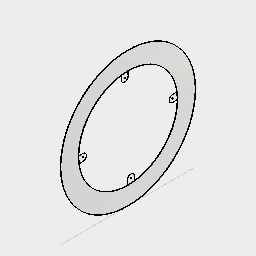
base (Autodesk Fusion 360 design; units mm, degrees)
Autodesk Fusion 360 part; units mm, degrees
note: some values were not read from the file. Set by a fixed rule: which sketch regions a step uses.
sketch "Sketch1" plane through (0, 0, 0) normal (1, 0, 0) x (0, 0, -1)
  circle A0 centre (0, 0) radius 381
  circle A1 centre (0, 0) radius 330.2
  dimension "d1" = 762
  dimension "d2" = 660.4
  measures "d1" diameter of A0
  measures "d2" diameter of A1
sketch "Sketch1 (2)" plane through (0, 0, 0) normal (1, 0, 0) x (0, 0, -1) in component "outer ring"
  circle A0 centre (0, 0) radius 381
  circle A1 centre (0, 0) radius 368.3
  dimension "d15" = 762
  dimension "d16" = 736.6
  measures "d15" diameter of A0
  measures "d16" diameter of A1
extrude "Extrude1" add sketch "Sketch1 (2)" along normal blind 6.35 makes body 1 in component "outer ring"
sketch "Sketch1 (3)" plane through (0, 0, 0) normal (1, 0, 0) x (0, 0, -1) in component "Top"
  circle A0 centre (0, 0) radius 381
  circle A1 centre (0, 0) radius 330.2
  dimension "d19" = 762
  dimension "d20" = 660.4
  measures "d19" diameter of A0
  measures "d20" diameter of A1
extrude "Extrude1'" add sketch "Sketch1 (3)" along normal blind 3.175 separate body makes body 2 in component "Top"
sketch "Sketch1 (4)" plane through (0, 0, 0) normal (1, 0, 0) x (0, 0, -1) in component "magnets"
  line L0 (-82.7081, 358.8931) -> (-70.2852, 361.5313)
  line L1 (-70.2852, 361.5313) -> (-67.647, 349.1083)
  line L2 (-67.647, 349.1083) -> (-80.0699, 346.4701)
  line L3 (-80.0699, 346.4701) -> (-82.7081, 358.8931)
  circle A0 centre (0, 0) radius 368.3
  line L4 (-82.7081, 358.8931) -> (-70.2852, 361.5313)
  dimension "d23" = 12.7
  dimension "d24" = 12.7
  measures "d23" distance of L0.start L0.end
  measures "d24" distance of L0.start L2.end
extrude "Extrude1''" add sketch "Sketch1 (4)" along normal blind 6.35 separate body contours L0 L1 L2 L3 L4 makes body 3 in component "magnets"
pattern_circular "C-Pattern1" count 176 over 360 about axis through (6.35, 0, 0) along (-1, 0, 0) of bodies 3 makes body 4 at (0, 358.1778, 64.9449) makes body 5 at (0, 356.6562, 47.3444) makes body 6 at (0, 358.1187, 34.5844) makes body 7 at (0, 363.0678, 26.2854) makes body 8 at (0, 363.7747, 13.3099) makes body 9 at (0, 364.0179, 0.3174) makes body 10 at (0, 363.7973, -12.6754) makes body 11 at (0, 363.1131, -25.6521) makes body 12 at (0, 357.286, -42.3296) makes body 13 at (0, 360.3579, -51.4909) makes body 14 at (0, 353.356, -67.7102) makes body 15 at (0, 350.7141, -80.2792) makes body 16 at (0, 347.6253, -92.7458) makes body 17 at (0, 344.0934, -105.0943) makes body 18 at (0, 340.1231, -117.3088) makes body 19 at (0, 341.1774, -126.9138) makes body 20 at (0, 336.4302, -139.0104) makes body 21 at (0, 325.6346, -152.9942) makes body 22 at (0, 319.9664, -164.5194) makes body 23 at (0, 319.643, -174.1766) makes body 24 at (0, 313.2226, -185.4744) makes body 25 at (0, 300.5468, -197.7796) makes body 26 at (0, 299.1929, -207.3469) makes body 27 at (0, 291.6016, -217.8937) makes body 28 at (0, 277.683, -228.7733) makes body 29 at (0, 269.3407, -238.5387) makes body 30 at (0, 260.655, -248.0001) makes body 31 at (0, 257.624, -257.1751) makes body 32 at (0, 242.2988, -265.9632) makes body 33 at (0, 238.621, -274.8985) makes body 34 at (0, 222.7078, -282.5709) makes body 35 at (0, 218.4019, -291.2211) makes body 36 at (0, 207.8684, -298.8309) makes body 37 at (0, 191.2263, -304.7583) makes body 38 at (0, 186.0204, -312.8986) makes body 39 at (0, 174.7338, -319.3388) makes body 40 at (0, 157.5535, -323.4533) makes body 41 at (0, 145.9083, -328.8706) makes body 42 at (0, 134.0772, -333.8689) makes body 43 at (0, 127.5087, -340.9556) makes body 44 at (0, 115.2579, -345.2894) makes body 45 at (0, 97.62, -346.2881) makes body 46 at (0, 90.3316, -352.6321) makes body 47 at (0, 72.6674, -352.3699) makes body 48 at (0, 64.9449, -358.1778) makes body 49 at (0, 47.3444, -356.6562) makes body 50 at (0, 39.2274, -361.8983) makes body 51 at (0, 26.2854, -363.0678) makes body 52 at (0, 13.3099, -363.7747) makes body 53 at (0, -3.8949, -359.7637) makes body 54 at (0, -12.6754, -363.7973) makes body 55 at (0, -25.6521, -363.1131) makes body 56 at (0, -42.3296, -357.286) makes body 57 at (0, -51.4909, -360.3579) makes body 58 at (0, -64.3202, -358.2905) makes body 59 at (0, -77.0674, -355.7665) makes body 60 at (0, -92.7458, -347.6253) makes body 61 at (0, -102.2511, -349.3621) makes body 62 at (0, -117.3088, -340.1231) makes body 63 at (0, -129.3739, -335.7194) makes body 64 at (0, -141.2741, -330.8878) makes body 65 at (0, -152.9942, -325.6346) makes body 66 at (0, -162.6568, -325.6561) makes body 67 at (0, -175.8349, -313.8904) makes body 68 at (0, -185.4744, -313.2226) makes body 69 at (0, -197.7796, -300.5468) makes body 70 at (0, -208.3808, -293.296) makes body 71 at (0, -218.7164, -285.6716) makes body 72 at (0, -228.1628, -283.6387) makes body 73 at (0, -238.5387, -269.3407) makes body 74 at (0, -247.816, -266.639) makes body 75 at (0, -257.1751, -257.624) makes body 76 at (0, -266.2064, -248.2807) makes body 77 at (0, -274.4419, -232.6516) makes body 78 at (0, -282.5709, -222.7078) makes body 79 at (0, -290.3398, -212.4803) makes body 80 at (0, -298.8309, -207.8684) makes body 81 at (0, -304.7583, -191.2263) makes body 82 at (0, -311.3894, -180.227) makes body 83 at (0, -317.6237, -168.9979) makes body 84 at (0, -323.4533, -157.5535) makes body 85 at (0, -330.9905, -151.5073) makes body 86 at (0, -336.1872, -139.5969) makes body 87 at (0, -338.4417, -122.0752) makes body 88 at (0, -345.2894, -115.2579) makes body 89 at (0, -346.2881, -97.62) makes body 90 at (0, -352.6321, -90.3316) makes body 91 at (0, -352.3699, -72.6674) makes body 92 at (0, -358.1778, -64.9449) makes body 93 at (0, -356.6562, -47.3444) makes body 94 at (0, -361.8983, -39.2274) makes body 95 at (0, -363.0678, -26.2854) makes body 96 at (0, -363.7747, -13.3099) makes body 97 at (0, -364.0179, -0.3174) makes body 98 at (0, -363.7973, 12.6754) makes body 99 at (0, -363.1131, 25.6521) makes body 100 at (0, -361.9662, 38.5961) makes body 101 at (0, -360.3579, 51.4909) makes body 102 at (0, -358.2905, 64.3202) makes body 103 at (0, -350.7141, 80.2792) makes body 104 at (0, -347.6253, 92.7458) makes body 105 at (0, -349.3621, 102.2511) makes body 106 at (0, -345.4899, 114.6555) makes body 107 at (0, -341.1774, 126.9138) makes body 108 at (0, -330.8878, 141.2741) makes body 109 at (0, -325.6346, 152.9942) makes body 110 at (0, -325.6561, 162.6568) makes body 111 at (0, -319.643, 174.1766) makes body 112 at (0, -313.2226, 185.4744) makes body 113 at (0, -306.403, 196.5359) makes body 114 at (0, -299.1929, 207.3469) makes body 115 at (0, -285.6716, 218.7164) makes body 116 at (0, -283.6387, 228.1628) makes body 117 at (0, -275.3143, 238.1412) makes body 118 at (0, -260.655, 248.0001) makes body 119 at (0, -251.6372, 257.1455) makes body 120 at (0, -242.2988, 265.9632) makes body 121 at (0, -238.621, 274.8985) makes body 122 at (0, -228.6571, 283.2403) makes body 123 at (0, -218.4019, 291.2211) makes body 124 at (0, -207.8684, 298.8309) makes body 125 at (0, -191.2263, 304.7583) makes body 126 at (0, -186.0204, 312.8986) makes body 127 at (0, -174.7338, 319.3388) makes body 128 at (0, -157.5535, 323.4533) makes body 129 at (0, -151.5073, 330.9905) makes body 130 at (0, -134.0772, 333.8689) makes body 131 at (0, -127.5087, 340.9556) makes body 132 at (0, -115.2579, 345.2894) makes body 133 at (0, -97.62, 346.2881) makes body 134 at (0, -90.3316, 352.6321) makes body 135 at (0, -77.6878, 355.6315) makes body 136 at (0, -64.9449, 358.1778) makes body 137 at (0, -47.3444, 356.6562) makes body 138 at (0, -39.2274, 361.8983) makes body 139 at (0, -26.2854, 363.0678) makes body 140 at (0, -13.3099, 363.7747) makes body 141 at (0, -0.3174, 364.0179) makes body 142 at (0, 12.6754, 363.7973) makes body 143 at (0, 25.6521, 363.1131) makes body 144 at (0, 38.5961, 361.9662) makes body 145 at (0, 51.4909, 360.3579) makes body 146 at (0, 64.3202, 358.2905) makes body 147 at (0, 80.2792, 350.7141) makes body 148 at (0, 92.7458, 347.6253) makes body 149 at (0, 105.0943, 344.0934) makes body 150 at (0, 117.3088, 340.1231) makes body 151 at (0, 129.3739, 335.7194) makes body 152 at (0, 141.2741, 330.8878) makes body 153 at (0, 150.9298, 331.2542) makes body 154 at (0, 162.6568, 325.6561) makes body 155 at (0, 174.1766, 319.643) makes body 156 at (0, 185.4744, 313.2226) makes body 157 at (0, 197.7796, 300.5468) makes body 158 at (0, 207.3469, 299.1929) makes body 159 at (0, 217.8937, 291.6016) makes body 160 at (0, 228.1628, 283.6387) makes body 161 at (0, 238.1412, 275.3143) makes body 162 at (0, 247.816, 266.639) makes body 163 at (0, 257.1455, 251.6372) makes body 164 at (0, 265.9632, 242.2988) makes body 165 at (0, 274.8985, 238.621) makes body 166 at (0, 283.2403, 228.6571) makes body 167 at (0, 291.2211, 218.4019) makes body 168 at (0, 297.7388, 201.982) makes body 169 at (0, 306.0598, 197.07) makes body 170 at (0, 312.8986, 186.0204) makes body 171 at (0, 319.3388, 174.7338) makes body 172 at (0, 323.4533, 157.5535) makes body 173 at (0, 330.9905, 151.5073) makes body 174 at (0, 333.8689, 134.0772) makes body 175 at (0, 338.4417, 122.0752) makes body 176 at (0, 342.5832, 109.9176) makes body 177 at (0, 349.1832, 102.8603) makes body 178 at (0, 352.6321, 90.3316) in component "magnets"
sketch "Sketch1 (5)" plane through (0, 0, 0) normal (1, 0, 0) x (0, 0, -1) in component "middle ring"
  circle A0 centre (0, 0) radius 354.965
  circle A1 centre (0, 0) radius 342.265
  dimension "d29" = 709.93
  dimension "d30" = 12.7
  measures "d29" diameter of A0
extrude "Extrude1'''" add sketch "Sketch1 (5)" along normal blind 6.35 separate body makes body 179 in component "middle ring"
sketch "Sketch2" plane through (0, 0, 0) normal (1, 0, 0) x (0, 0, -1) in component "magnets"
  circle A0 centre (0, 0) radius 342.265
  line L0 (-28.5855, 341.0692) -> (-15.9123, 341.8949)
  line L1 (-15.9123, 341.8949) -> (-15.0866, 329.2218)
  line L2 (-15.0866, 329.2218) -> (-27.7598, 328.3961)
  line L3 (-27.7598, 328.3961) -> (-28.5855, 341.0692)
  dimension "d35" = 12.7
  dimension "d36" = 12.7
  measures "d35" distance of L0.start L0.end
  measures "d36" distance of L0.start L2.end
extrude "Extrude2" add sketch "Sketch2" along normal blind 6.35 separate body contours L0 L1 L2 L3 makes body 180 in component "magnets"
pattern_circular "C-Pattern2" count 163 over 360 about axis through (6.35, 0, 0) along (-1, 0, 0) of bodies 180 makes body 181 at (0, 333.566, 10.9639) makes body 182 at (0, 333.7407, -1.899) makes body 183 at (0, 333.4196, -14.7592) makes body 184 at (0, 332.6032, -27.5974) makes body 185 at (0, 331.2926, -40.3947) makes body 186 at (0, 329.4897, -53.1319) makes body 187 at (0, 327.1974, -65.7901) makes body 188 at (0, 324.4189, -78.3507) makes body 189 at (0, 321.1585, -90.7948) makes body 190 at (0, 317.4209, -103.104) makes body 191 at (0, 313.2117, -115.2601) makes body 192 at (0, 308.5372, -127.2449) makes body 193 at (0, 303.4043, -139.0407) makes body 194 at (0, 297.8206, -150.6298) makes body 195 at (0, 291.7945, -161.9952) makes body 196 at (0, 285.3348, -173.12) makes body 197 at (0, 278.4512, -183.9875) makes body 198 at (0, 271.1539, -194.5817) makes body 199 at (0, 263.4538, -204.8867) makes body 200 at (0, 255.8378, -220.8553) makes body 201 at (0, 246.8913, -224.5688) makes body 202 at (0, 238.0536, -233.9166) makes body 203 at (0, 228.8621, -242.9169) makes body 204 at (0, 219.3307, -251.5562) makes body 205 at (0, 209.4734, -259.8218) makes body 206 at (0, 199.3049, -267.7014) makes body 207 at (0, 188.8403, -275.1833) makes body 208 at (0, 178.0951, -282.2563) makes body 209 at (0, 167.0853, -288.91) makes body 210 at (0, 155.8273, -295.1345) makes body 211 at (0, 142.3158, -306.5555) makes body 212 at (0, 132.6338, -306.2593) makes body 213 at (0, 118.2828, -316.6058) makes body 214 at (0, 108.6523, -315.5648) makes body 215 at (0, 96.4105, -319.5176) makes body 216 at (0, 84.0255, -322.9957) makes body 217 at (0, 68.2558, -331.0154) makes body 218 at (0, 58.8994, -328.5078) makes body 219 at (0, 42.5589, -335.2891) makes body 220 at (0, 33.4235, -332.0683) makes body 221 at (0, 20.6015, -333.1097) makes body 222 at (0, 7.749, -333.6562) makes body 223 at (0, -5.1151, -333.7069) makes body 224 at (0, -17.9716, -333.2619) makes body 225 at (0, -30.8013, -332.3218) makes body 226 at (0, -43.5853, -330.8879) makes body 227 at (0, -56.3046, -328.9624) makes body 228 at (0, -68.9402, -326.5482) makes body 229 at (0, -81.4733, -323.6488) makes body 230 at (0, -93.8855, -320.2686) makes body 231 at (0, -106.1581, -316.4126) makes body 232 at (0, -118.273, -312.0865) makes body 233 at (0, -135.7759, -309.5076) makes body 234 at (0, -141.958, -302.0503) makes body 235 at (0, -153.4928, -296.3552) makes body 236 at (0, -164.7996, -290.2198) makes body 237 at (0, -175.8616, -283.6533) makes body 238 at (0, -186.6623, -276.6653) makes body 239 at (0, -197.1856, -269.2662) makes body 240 at (0, -207.416, -261.4672) makes body 241 at (0, -217.3383, -253.2796) makes body 242 at (0, -226.9376, -244.7158) makes body 243 at (0, -236.1998, -235.7883) makes body 244 at (0, -245.111, -226.5106) makes body 245 at (0, -253.6581, -216.8964) makes body 246 at (0, -267.7701, -206.2262) makes body 247 at (0, -269.6096, -196.7159) makes body 248 at (0, -276.9903, -186.1796) makes body 249 at (0, -289.7768, -173.9525) makes body 250 at (0, -290.5067, -164.2934) makes body 251 at (0, -296.6224, -152.9759) makes body 252 at (0, -302.2974, -141.4312) makes body 253 at (0, -307.5232, -129.6763) makes body 254 at (0, -317.731, -115.2263) makes body 255 at (0, -316.5972, -105.6063) makes body 256 at (0, -320.4318, -93.327) makes body 257 at (0, -323.7904, -80.909) makes body 258 at (0, -331.6578, -65.0627) makes body 259 at (0, -329.0601, -55.731) makes body 260 at (0, -330.9634, -43.0084) makes body 261 at (0, -332.375, -30.2219) makes body 262 at (0, -333.2927, -17.3905) makes body 263 at (0, -337.9792, -0.3307) makes body 264 at (0, -333.6421, 8.3307) makes body 265 at (0, -333.0733, 21.1822) makes body 266 at (0, -332.0095, 34.0024) makes body 267 at (0, -334.0204, 51.5795) makes body 268 at (0, -328.4046, 59.4721) makes body 269 at (0, -325.8687, 72.0838) makes body 270 at (0, -322.8487, 84.5885) makes body 271 at (0, -319.349, 96.9674) makes body 272 at (0, -315.3749, 109.2023) makes body 273 at (0, -310.9322, 121.275) makes body 274 at (0, -306.0276, 133.1675) makes body 275 at (0, -300.6683, 144.8622) makes body 276 at (0, -294.8623, 156.3416) makes body 277 at (0, -288.6183, 167.5887) makes body 278 at (0, -281.9454, 178.5869) makes body 279 at (0, -274.8536, 189.3197) makes body 280 at (0, -267.3535, 199.7713) makes body 281 at (0, -259.4562, 209.9261) makes body 282 at (0, -251.1734, 219.7689) makes body 283 at (0, -242.5175, 229.2853) makes body 284 at (0, -233.5012, 238.461) makes body 285 at (0, -224.1381, 247.2825) makes body 286 at (0, -214.4419, 255.7365) makes body 287 at (0, -204.4271, 263.8106) makes body 288 at (0, -194.1086, 271.4928) makes body 289 at (0, -182.2562, 284.6274) makes body 290 at (0, -172.6222, 285.6362) makes body 291 at (0, -161.4863, 292.0765) makes body 292 at (0, -150.1104, 298.0828) makes body 293 at (0, -138.5115, 303.6463) makes body 294 at (0, -126.7068, 308.7586) makes body 295 at (0, -112.1591, 318.8266) makes body 296 at (0, -102.5505, 317.6002) makes body 297 at (0, -90.2347, 321.3163) makes body 298 at (0, -77.785, 324.5551) makes body 299 at (0, -65.2196, 327.3116) makes body 300 at (0, -52.5573, 329.5819) makes body 301 at (0, -39.817, 331.3625) makes body 302 at (0, -27.0175, 332.6508) makes body 303 at (0, -14.1779, 333.4449) makes body 304 at (0, -1.3172, 333.7435) makes body 305 at (0, 11.5455, 333.5464) makes body 306 at (0, 24.391, 332.8537) makes body 307 at (0, 37.2002, 331.6664) makes body 308 at (0, 49.9542, 329.9865) makes body 309 at (0, 62.634, 327.8162) makes body 310 at (0, 75.2207, 325.1589) makes body 311 at (0, 87.6957, 322.0185) makes body 312 at (0, 100.0404, 318.3998) makes body 313 at (0, 112.2364, 314.3079) makes body 314 at (0, 124.2657, 309.7491) makes body 315 at (0, 136.1104, 304.7301) makes body 316 at (0, 147.7529, 299.2584) makes body 317 at (0, 159.1758, 293.342) makes body 318 at (0, 170.3623, 286.9899) makes body 319 at (0, 181.2956, 280.2113) makes body 320 at (0, 191.9596, 273.0165) makes body 321 at (0, 202.3384, 265.416) makes body 322 at (0, 212.4166, 257.4212) makes body 323 at (0, 222.1792, 249.0439) makes body 324 at (0, 231.6117, 240.2967) makes body 325 at (0, 240.7001, 231.1924) makes body 326 at (0, 249.4309, 221.7447) makes body 327 at (0, 257.7911, 211.9675) makes body 328 at (0, 271.6948, 201.0273) makes body 329 at (0, 273.3507, 191.4833) makes body 330 at (0, 280.527, 180.8068) makes body 331 at (0, 287.2864, 169.8617) makes body 332 at (0, 299.345, 156.916) makes body 333 at (0, 299.5155, 147.2309) makes body 334 at (0, 310.5412, 133.395) makes body 335 at (0, 309.9653, 123.7255) makes body 336 at (0, 314.5031, 111.6883) makes body 337 at (0, 318.5737, 99.4851) makes body 338 at (0, 322.171, 87.1341) makes body 339 at (0, 330.3423, 71.4425) makes body 340 at (0, 327.9249, 62.0624) makes body 341 at (0, 330.073, 49.3788) makes body 342 at (0, 331.7308, 36.6219) in component "magnets"
sketch "Sketch1 (6)" plane through (0, 0, 0) normal (1, 0, 0) x (0, 0, -1) in component "Inner ring"
  circle A0 centre (0, 0) radius 328.93
sketch "Sketch3" plane through (0, 0, 0) normal (1, 0, 0) x (0, 0, -1)
  circle A0 centre (0, 0) radius 381
  circle A1 centre (0, 0) radius 279.4
  dimension "d49" = 762
  dimension "d50" = 558.8
  measures "d49" diameter of A0
  measures "d50" diameter of A1
extrude "Extrude5" add sketch "Sketch3" along normal blind 1.524 separate body makes body 343
sketch "Sketch4" plane through (0, 0, 0) normal (1, 0, 0) x (0, 0, -1)
  line L0 (-279.4, 0) -> (-276.8023, -38.0113)
  line L1 (-276.8023, -38.0113) -> (-251.4614, -36.2795)
  line L2 (-251.4614, -36.2795) -> (-254.0591, 1.7318)
  line L3 (-254.0591, 1.7318) -> (-279.4, 0)
  circle A0 centre (0, 0) radius 279.4
  circle A1 centre (-252.7602, -17.2739) radius 19.05
  point P0 (-279.4, 0)
  dimension "d53" = 38.1
  dimension "d54" = 25.4
  dimension "d55" = 38.1
  measures "d53" distance of P0 L0.end
  measures "d54" distance of P0 L2.end
  measures "d55" diameter of A1
extrude "Extrude6" add sketch "Sketch4" along normal blind 25.4 separate body contours L0 L1 L3 A1 | L2 A1 | L2 A1 makes body 344
hole "Hole2" at (25.4, -17.2739, 252.7602) direction (-1, 0, 0) diameter 6.604 depth 25.4 tip angle 118 bodies 344
pattern_circular "C-Pattern2'" count 4 over 360 about axis through (1.524, 0, 0) along (-1, 0, 0) of bodies 344 makes body 345 at (16.9333, 244.1809, 34.2826) makes body 346 at (16.9333, 34.2826, -244.1809) makes body 347 at (16.9333, -246.8118, -35.3713)
extrude "Extrude7" cut 1 faces at (25.4, -18.4284, 270.7548) along direction (-1, 0, 0) blind 23.876 on bodies 344 bodies 344
extrude "Extrude8" add 1 faces at (0.508, -12.6704, 278.5341) along direction (0, -0.068182, 0.997673) blind 5.08 on bodies 344 bodies 344 345 346 347 343
extrude "Extrude9" cut 1 faces at (25.4, 270.7548, 18.4284) along direction (-1, 0, 0) blind 23.876 on bodies 345 bodies 345
extrude "Extrude10" add 1 faces at (0.508, 278.5341, 12.6704) along direction (0, 0.997673, 0.068182) blind 5.08 on bodies 345 bodies 345 346 347 344
extrude "Extrude11" cut 1 faces at (25.4, -270.7548, -18.4284) along direction (-1, 0, 0) blind 23.876 on bodies 347 bodies 347
extrude "Extrude12" add 1 faces at (1.016, -278.5341, -12.6704) along direction (0, -0.997673, -0.068182) blind 5.08 on bodies 347 bodies 347 346 345
extrude "Extrude13" cut 1 faces at (25.4, 18.4284, -270.7548) along direction (-1, 0, 0) blind 23.876 on bodies 346 bodies 346
extrude "Extrude14" add 1 faces at (1.016, 12.6704, -278.5341) along direction (0, 0.068182, -0.997673) blind 5.08 on bodies 346 bodies 346 347
sketch "Sketch2 (2)" plane through (0, 0, 0) normal (1, 0, 0) x (0, 0, -1) in component "Top"
  circle A0 centre (0, 0) radius 279.4
  circle A1 centre (0, 0) radius 330.2
  dimension "d80" = 558.8
  dimension "d81" = 660.4
  measures "d80" diameter of A0
  measures "d81" diameter of A1
extrude "Extrude2'" add sketch "Sketch2 (2)" along normal blind 3.175 bodies 2 in component "Top"
sketch "Sketch2 (3)" plane through (0, 0, 0) normal (1, 0, 0) x (0, 0, -1) in component "Inner ring"
  circle A0 centre (0, 0) radius 279.4
  circle A1 centre (0, 0) radius 329.565
  dimension "d84" = 558.8
  dimension "d85" = 659.13
  measures "d84" diameter of A0
  measures "d85" diameter of A1
extrude "Extrude1''''" add sketch "Sketch1 (6)" along normal blind 6.35 separate body makes body 348 in component "Inner ring"
extrude "Extrude2''" cut sketch "Sketch2 (3)" along normal blind 6.35 contours A0 bodies 348 in component "Inner ring"
sketch "Sketch3 (2)" plane through (0, 0, 0) normal (1, 0, 0) x (0, 0, -1) in component "Top"
  circle A0 centre (0, 0) radius 381
  line L0 (0, 0) -> (-505.5205, -34.5477) construction
  line L1 (0, 0) -> (-394.1153, 343.6928) construction
  circle A1 centre (0, 0) radius 304.8 construction
  arc A2 (-251.4614, -36.2795) -> (-254.0591, 1.7318) centre (-252.7602, -17.2739) ccw
  circle A3 centre (-229.7196, 200.3296) radius 3.302
  circle A4 centre (0, 0) radius 349.25 construction
  circle A5 centre (0, 0) radius 374.65 construction
  circle A6 centre (-263.2203, 229.5444) radius 3.302
  line L2 (0, 0) -> (361.2841, 414.2873) construction
  line L3 (0, 0) -> (437.0322, -381.1191) construction
  line L4 (0, 0) -> (-358.3327, -410.903) construction
  circle A7 centre (-282.3636, 246.2385) radius 3.302
  dimension "d94" = 45
  dimension "d95" = 609.6
  dimension "d96" = 6.604
  dimension "d103" = 698.5
  dimension "d105" = 749.3
  dimension "d113" = 6.604
  dimension "d127" = 90
  dimension "d129" = 90
  dimension "d130" = 90
  dimension "d140" = 6.604
  measures "d94" angle of L0 L1
  measures "d95" diameter of A1
  measures "d96" diameter of A3
  measures "d103" diameter of A4
  measures "d105" diameter of A5
  measures "d113" diameter of A6
  measures "d127" angle of L1 L2
  measures "d129" angle of L2 L3
  measures "d130" angle of L3 L4
  measures "d140" diameter of A7
extrude "Extrude19" [suppressed]
extrude "Extrude17" [suppressed]
extrude "Extrude16" [suppressed]
extrude "Extrude15" [suppressed]
sketch "Sketch4 (2)" plane through (-7.874, 0, 0) normal (-1, 0, 0) x (0, 0, 1) in component "Top"
  circle A0 centre (229.7196, 200.3296) radius 3.302
  circle A1 centre (263.2203, 229.5444) radius 3.302
  circle A2 centre (0, 0) radius 381
  circle A3 centre (252.7602, -17.2739) radius 3.302
  circle A4 centre (17.2739, 252.7602) radius 3.302
  circle A5 centre (-17.2739, -252.7602) radius 3.302
  line L0 (-279.4, 0) -> (-254.0591, -1.7318)
  arc A6 (-254.0591, -1.7318) -> (-251.4614, 36.2795) centre (-252.7602, 17.2739) ccw
  line L1 (-251.4614, 36.2795) -> (-276.8023, 38.0113)
  arc A7 (0, 279.4) -> (-276.8023, 38.0113) centre (0, 0) ccw
  line L2 (0, 279.4) -> (-1.7318, 254.0591)
  arc A8 (-1.7318, 254.0591) -> (36.2795, 251.4614) centre (17.2739, 252.7602) ccw
  line L3 (36.2795, 251.4614) -> (38.0113, 276.8023)
  arc A9 (279.4, 0) -> (38.0113, 276.8023) centre (0, 0) ccw
  line L4 (279.4, 0) -> (254.0591, 1.7318)
  arc A10 (254.0591, 1.7318) -> (251.4614, -36.2795) centre (252.7602, -17.2739) ccw
  line L5 (251.4614, -36.2795) -> (276.8023, -38.0113)
  arc A11 (0, -279.4) -> (276.8023, -38.0113) centre (0, 0) ccw
  line L6 (0, -279.4) -> (1.7318, -254.0591)
  arc A12 (1.7318, -254.0591) -> (-36.2795, -251.4614) centre (-17.2739, -252.7602) ccw
  line L7 (-36.2795, -251.4614) -> (-38.0113, -276.8023)
  arc A13 (-279.4, 0) -> (-38.0113, -276.8023) centre (0, 0) ccw
  circle A14 centre (-252.7602, 17.2739) radius 3.302
  circle A15 centre (282.3636, 246.2385) radius 3.302
  line L8 (0, 0) -> (394.1153, 343.6928)
  circle A16 centre (0, 0) radius 374.65
  circle A17 centre (282.3636, 246.2385) radius 3.302
  dimension "d120" = 6.604
  measures "d120" diameter of A15
extrude "Extrude18" [suppressed]
sketch "Sketch5" plane through (-7.874, 0, 0) normal (-1, 0, 0) x (0, 0, 1) in component "Top"
  circle A0 centre (229.7196, 200.3296) radius 3.302
  circle A1 centre (263.2203, 229.5444) radius 3.302
  circle A2 centre (282.3636, 246.2385) radius 3.302
  circle A3 centre (0, 0) radius 381
  circle A4 centre (252.7602, -17.2739) radius 3.302
  circle A5 centre (17.2739, 252.7602) radius 3.302
  circle A6 centre (-17.2739, -252.7602) radius 3.302
  line L0 (-279.4, 0) -> (-254.0591, -1.7318)
  arc A7 (-254.0591, -1.7318) -> (-251.4614, 36.2795) centre (-252.7602, 17.2739) ccw
  line L1 (-251.4614, 36.2795) -> (-276.8023, 38.0113)
  arc A8 (0, 279.4) -> (-276.8023, 38.0113) centre (0, 0) ccw
  line L2 (0, 279.4) -> (-1.7318, 254.0591)
  arc A9 (-1.7318, 254.0591) -> (36.2795, 251.4614) centre (17.2739, 252.7602) ccw
  line L3 (36.2795, 251.4614) -> (38.0113, 276.8023)
  arc A10 (279.4, 0) -> (38.0113, 276.8023) centre (0, 0) ccw
  line L4 (279.4, 0) -> (254.0591, 1.7318)
  arc A11 (254.0591, 1.7318) -> (251.4614, -36.2795) centre (252.7602, -17.2739) ccw
  line L5 (251.4614, -36.2795) -> (276.8023, -38.0113)
  arc A12 (0, -279.4) -> (276.8023, -38.0113) centre (0, 0) ccw
  line L6 (0, -279.4) -> (1.7318, -254.0591)
  arc A13 (1.7318, -254.0591) -> (-36.2795, -251.4614) centre (-17.2739, -252.7602) ccw
  line L7 (-36.2795, -251.4614) -> (-38.0113, -276.8023)
  arc A14 (-279.4, 0) -> (-38.0113, -276.8023) centre (0, 0) ccw
  circle A15 centre (-252.7602, 17.2739) radius 3.302
  circle A16 centre (-246.2385, 282.3636) radius 3.302
  line L8 (0, 0) -> (-361.2841, 414.2873)
  circle A17 centre (0, 0) radius 374.65
  dimension "d147" = 6.604
  measures "d147" diameter of A16
extrude "Extrude20" [suppressed]
sketch "Sketch6" plane through (-7.874, 0, 0) normal (-1, 0, 0) x (0, 0, 1) in component "Top"
  circle A0 centre (-246.2385, 282.3636) radius 3.302
  circle A1 centre (229.7196, 200.3296) radius 3.302
  circle A2 centre (263.2203, 229.5444) radius 3.302
  circle A3 centre (282.3636, 246.2385) radius 3.302
  circle A4 centre (0, 0) radius 381
  circle A5 centre (252.7602, -17.2739) radius 3.302
  circle A6 centre (17.2739, 252.7602) radius 3.302
  circle A7 centre (-17.2739, -252.7602) radius 3.302
  line L0 (-279.4, 0) -> (-254.0591, -1.7318)
  arc A8 (-254.0591, -1.7318) -> (-251.4614, 36.2795) centre (-252.7602, 17.2739) ccw
  line L1 (-251.4614, 36.2795) -> (-276.8023, 38.0113)
  arc A9 (0, 279.4) -> (-276.8023, 38.0113) centre (0, 0) ccw
  line L2 (0, 279.4) -> (-1.7318, 254.0591)
  arc A10 (-1.7318, 254.0591) -> (36.2795, 251.4614) centre (17.2739, 252.7602) ccw
  line L3 (36.2795, 251.4614) -> (38.0113, 276.8023)
  arc A11 (279.4, 0) -> (38.0113, 276.8023) centre (0, 0) ccw
  line L4 (279.4, 0) -> (254.0591, 1.7318)
  arc A12 (254.0591, 1.7318) -> (251.4614, -36.2795) centre (252.7602, -17.2739) ccw
  line L5 (251.4614, -36.2795) -> (276.8023, -38.0113)
  arc A13 (0, -279.4) -> (276.8023, -38.0113) centre (0, 0) ccw
  line L6 (0, -279.4) -> (1.7318, -254.0591)
  arc A14 (1.7318, -254.0591) -> (-36.2795, -251.4614) centre (-17.2739, -252.7602) ccw
  line L7 (-36.2795, -251.4614) -> (-38.0113, -276.8023)
  arc A15 (-279.4, 0) -> (-38.0113, -276.8023) centre (0, 0) ccw
  circle A16 centre (-252.7602, 17.2739) radius 3.302
  circle A17 centre (-229.5444, 263.2203) radius 3.302
  line L8 (0, 0) -> (-361.2841, 414.2873)
  circle A18 centre (0, 0) radius 349.25
  dimension "d154" = 6.604
  measures "d154" diameter of A17
extrude "Extrude21" [suppressed]
sketch "Sketch7" plane through (-7.874, 0, 0) normal (-1, 0, 0) x (0, 0, 1) in component "Top"
  circle A0 centre (-229.5444, 263.2203) radius 3.302
  circle A1 centre (-246.2385, 282.3636) radius 3.302
  circle A2 centre (229.7196, 200.3296) radius 3.302
  circle A3 centre (263.2203, 229.5444) radius 3.302
  circle A4 centre (282.3636, 246.2385) radius 3.302
  circle A5 centre (0, 0) radius 381
  circle A6 centre (252.7602, -17.2739) radius 3.302
  circle A7 centre (17.2739, 252.7602) radius 3.302
  circle A8 centre (-17.2739, -252.7602) radius 3.302
  line L0 (-279.4, 0) -> (-254.0591, -1.7318)
  arc A9 (-254.0591, -1.7318) -> (-251.4614, 36.2795) centre (-252.7602, 17.2739) ccw
  line L1 (-251.4614, 36.2795) -> (-276.8023, 38.0113)
  arc A10 (0, 279.4) -> (-276.8023, 38.0113) centre (0, 0) ccw
  line L2 (0, 279.4) -> (-1.7318, 254.0591)
  arc A11 (-1.7318, 254.0591) -> (36.2795, 251.4614) centre (17.2739, 252.7602) ccw
  line L3 (36.2795, 251.4614) -> (38.0113, 276.8023)
  arc A12 (279.4, 0) -> (38.0113, 276.8023) centre (0, 0) ccw
  line L4 (279.4, 0) -> (254.0591, 1.7318)
  arc A13 (254.0591, 1.7318) -> (251.4614, -36.2795) centre (252.7602, -17.2739) ccw
  line L5 (251.4614, -36.2795) -> (276.8023, -38.0113)
  arc A14 (0, -279.4) -> (276.8023, -38.0113) centre (0, 0) ccw
  line L6 (0, -279.4) -> (1.7318, -254.0591)
  arc A15 (1.7318, -254.0591) -> (-36.2795, -251.4614) centre (-17.2739, -252.7602) ccw
  line L7 (-36.2795, -251.4614) -> (-38.0113, -276.8023)
  arc A16 (-279.4, 0) -> (-38.0113, -276.8023) centre (0, 0) ccw
  circle A17 centre (-252.7602, 17.2739) radius 3.302
  circle A18 centre (-200.3296, 229.7196) radius 3.302
  line L8 (0, 0) -> (-361.2841, 414.2873)
  circle A19 centre (0, 0) radius 304.8
  dimension "d161" = 6.604
  measures "d161" diameter of A18
extrude "Extrude22" [suppressed]
sketch "Sketch8" plane through (-7.874, 0, 0) normal (-1, 0, 0) x (0, 0, 1) in component "Top"
  circle A0 centre (-200.3296, 229.7196) radius 3.302
  circle A1 centre (-229.5444, 263.2203) radius 3.302
  circle A2 centre (-246.2385, 282.3636) radius 3.302
  circle A3 centre (229.7196, 200.3296) radius 3.302
  circle A4 centre (263.2203, 229.5444) radius 3.302
  circle A5 centre (282.3636, 246.2385) radius 3.302
  circle A6 centre (0, 0) radius 381
  circle A7 centre (252.7602, -17.2739) radius 3.302
  circle A8 centre (17.2739, 252.7602) radius 3.302
  circle A9 centre (-17.2739, -252.7602) radius 3.302
  line L0 (-279.4, 0) -> (-254.0591, -1.7318)
  arc A10 (-254.0591, -1.7318) -> (-251.4614, 36.2795) centre (-252.7602, 17.2739) ccw
  line L1 (-251.4614, 36.2795) -> (-276.8023, 38.0113)
  arc A11 (0, 279.4) -> (-276.8023, 38.0113) centre (0, 0) ccw
  line L2 (0, 279.4) -> (-1.7318, 254.0591)
  arc A12 (-1.7318, 254.0591) -> (36.2795, 251.4614) centre (17.2739, 252.7602) ccw
  line L3 (36.2795, 251.4614) -> (38.0113, 276.8023)
  arc A13 (279.4, 0) -> (38.0113, 276.8023) centre (0, 0) ccw
  line L4 (279.4, 0) -> (254.0591, 1.7318)
  arc A14 (254.0591, 1.7318) -> (251.4614, -36.2795) centre (252.7602, -17.2739) ccw
  line L5 (251.4614, -36.2795) -> (276.8023, -38.0113)
  arc A15 (0, -279.4) -> (276.8023, -38.0113) centre (0, 0) ccw
  line L6 (0, -279.4) -> (1.7318, -254.0591)
  arc A16 (1.7318, -254.0591) -> (-36.2795, -251.4614) centre (-17.2739, -252.7602) ccw
  line L7 (-36.2795, -251.4614) -> (-38.0113, -276.8023)
  arc A17 (-279.4, 0) -> (-38.0113, -276.8023) centre (0, 0) ccw
  circle A18 centre (-252.7602, 17.2739) radius 3.302
  circle A19 centre (-282.3636, -246.2385) radius 3.302
  line L8 (0, 0) -> (-437.0322, -381.1191)
  circle A20 centre (0, 0) radius 374.65
  dimension "d168" = 6.604
  measures "d168" diameter of A19
extrude "Extrude23" [suppressed]
sketch "Sketch9" plane through (-7.874, 0, 0) normal (-1, 0, 0) x (0, 0, 1) in component "Top"
  circle A0 centre (-282.3636, -246.2385) radius 3.302
  circle A1 centre (-200.3296, 229.7196) radius 3.302
  circle A2 centre (-229.5444, 263.2203) radius 3.302
  circle A3 centre (-246.2385, 282.3636) radius 3.302
  circle A4 centre (229.7196, 200.3296) radius 3.302
  circle A5 centre (263.2203, 229.5444) radius 3.302
  circle A6 centre (282.3636, 246.2385) radius 3.302
  circle A7 centre (0, 0) radius 381
  circle A8 centre (252.7602, -17.2739) radius 3.302
  circle A9 centre (17.2739, 252.7602) radius 3.302
  circle A10 centre (-17.2739, -252.7602) radius 3.302
  line L0 (-279.4, 0) -> (-254.0591, -1.7318)
  arc A11 (-254.0591, -1.7318) -> (-251.4614, 36.2795) centre (-252.7602, 17.2739) ccw
  line L1 (-251.4614, 36.2795) -> (-276.8023, 38.0113)
  arc A12 (0, 279.4) -> (-276.8023, 38.0113) centre (0, 0) ccw
  line L2 (0, 279.4) -> (-1.7318, 254.0591)
  arc A13 (-1.7318, 254.0591) -> (36.2795, 251.4614) centre (17.2739, 252.7602) ccw
  line L3 (36.2795, 251.4614) -> (38.0113, 276.8023)
  arc A14 (279.4, 0) -> (38.0113, 276.8023) centre (0, 0) ccw
  line L4 (279.4, 0) -> (254.0591, 1.7318)
  arc A15 (254.0591, 1.7318) -> (251.4614, -36.2795) centre (252.7602, -17.2739) ccw
  line L5 (251.4614, -36.2795) -> (276.8023, -38.0113)
  arc A16 (0, -279.4) -> (276.8023, -38.0113) centre (0, 0) ccw
  line L6 (0, -279.4) -> (1.7318, -254.0591)
  arc A17 (1.7318, -254.0591) -> (-36.2795, -251.4614) centre (-17.2739, -252.7602) ccw
  line L7 (-36.2795, -251.4614) -> (-38.0113, -276.8023)
  arc A18 (-279.4, 0) -> (-38.0113, -276.8023) centre (0, 0) ccw
  circle A19 centre (-252.7602, 17.2739) radius 3.302
  circle A20 centre (-263.2203, -229.5444) radius 3.302
  line L8 (0, 0) -> (-437.0322, -381.1191)
  circle A21 centre (0, 0) radius 349.25
  dimension "d175" = 6.604
  measures "d175" diameter of A20
extrude "Extrude24" [suppressed]
sketch "Sketch10" plane through (-7.874, 0, 0) normal (-1, 0, 0) x (0, 0, 1) in component "Top"
  circle A0 centre (-263.2203, -229.5444) radius 3.302
  circle A1 centre (-282.3636, -246.2385) radius 3.302
  circle A2 centre (-200.3296, 229.7196) radius 3.302
  circle A3 centre (-229.5444, 263.2203) radius 3.302
  circle A4 centre (-246.2385, 282.3636) radius 3.302
  circle A5 centre (229.7196, 200.3296) radius 3.302
  circle A6 centre (263.2203, 229.5444) radius 3.302
  circle A7 centre (282.3636, 246.2385) radius 3.302
  circle A8 centre (0, 0) radius 381
  circle A9 centre (252.7602, -17.2739) radius 3.302
  circle A10 centre (17.2739, 252.7602) radius 3.302
  circle A11 centre (-17.2739, -252.7602) radius 3.302
  line L0 (-279.4, 0) -> (-254.0591, -1.7318)
  arc A12 (-254.0591, -1.7318) -> (-251.4614, 36.2795) centre (-252.7602, 17.2739) ccw
  line L1 (-251.4614, 36.2795) -> (-276.8023, 38.0113)
  arc A13 (0, 279.4) -> (-276.8023, 38.0113) centre (0, 0) ccw
  line L2 (0, 279.4) -> (-1.7318, 254.0591)
  arc A14 (-1.7318, 254.0591) -> (36.2795, 251.4614) centre (17.2739, 252.7602) ccw
  line L3 (36.2795, 251.4614) -> (38.0113, 276.8023)
  arc A15 (279.4, 0) -> (38.0113, 276.8023) centre (0, 0) ccw
  line L4 (279.4, 0) -> (254.0591, 1.7318)
  arc A16 (254.0591, 1.7318) -> (251.4614, -36.2795) centre (252.7602, -17.2739) ccw
  line L5 (251.4614, -36.2795) -> (276.8023, -38.0113)
  arc A17 (0, -279.4) -> (276.8023, -38.0113) centre (0, 0) ccw
  line L6 (0, -279.4) -> (1.7318, -254.0591)
  arc A18 (1.7318, -254.0591) -> (-36.2795, -251.4614) centre (-17.2739, -252.7602) ccw
  line L7 (-36.2795, -251.4614) -> (-38.0113, -276.8023)
  arc A19 (-279.4, 0) -> (-38.0113, -276.8023) centre (0, 0) ccw
  circle A20 centre (-252.7602, 17.2739) radius 3.302
  circle A21 centre (-229.7196, -200.3296) radius 3.302
  circle A22 centre (0, 0) radius 304.8
  line L8 (0, 0) -> (-437.0322, -381.1191)
  dimension "d182" = 6.604
  measures "d182" diameter of A21
extrude "Extrude25" [suppressed]
sketch "Sketch11" plane through (-7.874, 0, 0) normal (-1, 0, 0) x (0, 0, 1) in component "Top"
  circle A0 centre (-229.7196, -200.3296) radius 3.302
  circle A1 centre (-263.2203, -229.5444) radius 3.302
  circle A2 centre (-282.3636, -246.2385) radius 3.302
  circle A3 centre (-200.3296, 229.7196) radius 3.302
  circle A4 centre (-229.5444, 263.2203) radius 3.302
  circle A5 centre (-246.2385, 282.3636) radius 3.302
  circle A6 centre (229.7196, 200.3296) radius 3.302
  circle A7 centre (263.2203, 229.5444) radius 3.302
  circle A8 centre (282.3636, 246.2385) radius 3.302
  circle A9 centre (0, 0) radius 381
  circle A10 centre (252.7602, -17.2739) radius 3.302
  circle A11 centre (17.2739, 252.7602) radius 3.302
  circle A12 centre (-17.2739, -252.7602) radius 3.302
  line L0 (-279.4, 0) -> (-254.0591, -1.7318)
  arc A13 (-254.0591, -1.7318) -> (-251.4614, 36.2795) centre (-252.7602, 17.2739) ccw
  line L1 (-251.4614, 36.2795) -> (-276.8023, 38.0113)
  arc A14 (0, 279.4) -> (-276.8023, 38.0113) centre (0, 0) ccw
  line L2 (0, 279.4) -> (-1.7318, 254.0591)
  arc A15 (-1.7318, 254.0591) -> (36.2795, 251.4614) centre (17.2739, 252.7602) ccw
  line L3 (36.2795, 251.4614) -> (38.0113, 276.8023)
  arc A16 (279.4, 0) -> (38.0113, 276.8023) centre (0, 0) ccw
  line L4 (279.4, 0) -> (254.0591, 1.7318)
  arc A17 (254.0591, 1.7318) -> (251.4614, -36.2795) centre (252.7602, -17.2739) ccw
  line L5 (251.4614, -36.2795) -> (276.8023, -38.0113)
  arc A18 (0, -279.4) -> (276.8023, -38.0113) centre (0, 0) ccw
  line L6 (0, -279.4) -> (1.7318, -254.0591)
  arc A19 (1.7318, -254.0591) -> (-36.2795, -251.4614) centre (-17.2739, -252.7602) ccw
  line L7 (-36.2795, -251.4614) -> (-38.0113, -276.8023)
  arc A20 (-279.4, 0) -> (-38.0113, -276.8023) centre (0, 0) ccw
  circle A21 centre (-252.7602, 17.2739) radius 3.302
  circle A22 centre (246.2385, -282.3636) radius 3.302
  circle A23 centre (0, 0) radius 374.65
  line L8 (0, 0) -> (358.3327, -410.903)
  dimension "d189" = 6.604
  measures "d189" diameter of A22
extrude "Extrude26" [suppressed]
sketch "Sketch12" plane through (-7.874, 0, 0) normal (-1, 0, 0) x (0, 0, 1) in component "Top"
  circle A0 centre (246.2385, -282.3636) radius 3.302
  circle A1 centre (-229.7196, -200.3296) radius 3.302
  circle A2 centre (-263.2203, -229.5444) radius 3.302
  circle A3 centre (-282.3636, -246.2385) radius 3.302
  circle A4 centre (-200.3296, 229.7196) radius 3.302
  circle A5 centre (-229.5444, 263.2203) radius 3.302
  circle A6 centre (-246.2385, 282.3636) radius 3.302
  circle A7 centre (229.7196, 200.3296) radius 3.302
  circle A8 centre (263.2203, 229.5444) radius 3.302
  circle A9 centre (282.3636, 246.2385) radius 3.302
  circle A10 centre (0, 0) radius 381
  circle A11 centre (252.7602, -17.2739) radius 3.302
  circle A12 centre (17.2739, 252.7602) radius 3.302
  circle A13 centre (-17.2739, -252.7602) radius 3.302
  line L0 (-279.4, 0) -> (-254.0591, -1.7318)
  arc A14 (-254.0591, -1.7318) -> (-251.4614, 36.2795) centre (-252.7602, 17.2739) ccw
  line L1 (-251.4614, 36.2795) -> (-276.8023, 38.0113)
  arc A15 (0, 279.4) -> (-276.8023, 38.0113) centre (0, 0) ccw
  line L2 (0, 279.4) -> (-1.7318, 254.0591)
  arc A16 (-1.7318, 254.0591) -> (36.2795, 251.4614) centre (17.2739, 252.7602) ccw
  line L3 (36.2795, 251.4614) -> (38.0113, 276.8023)
  arc A17 (279.4, 0) -> (38.0113, 276.8023) centre (0, 0) ccw
  line L4 (279.4, 0) -> (254.0591, 1.7318)
  arc A18 (254.0591, 1.7318) -> (251.4614, -36.2795) centre (252.7602, -17.2739) ccw
  line L5 (251.4614, -36.2795) -> (276.8023, -38.0113)
  arc A19 (0, -279.4) -> (276.8023, -38.0113) centre (0, 0) ccw
  line L6 (0, -279.4) -> (1.7318, -254.0591)
  arc A20 (1.7318, -254.0591) -> (-36.2795, -251.4614) centre (-17.2739, -252.7602) ccw
  line L7 (-36.2795, -251.4614) -> (-38.0113, -276.8023)
  arc A21 (-279.4, 0) -> (-38.0113, -276.8023) centre (0, 0) ccw
  circle A22 centre (-252.7602, 17.2739) radius 3.302
  circle A23 centre (229.5444, -263.2203) radius 3.302
  line L8 (0, 0) -> (358.3327, -410.903)
  circle A24 centre (0, 0) radius 349.25
  dimension "d196" = 6.604
  measures "d196" diameter of A23
extrude "Extrude27" [suppressed]
component "outer ring" placed x (1, 0, 0) y (0, 1, 0) z (0, 0, 1) at (1.524, 0, 0)
component "magnets" placed x (1, 0, 0) y (0, 1, 0) z (0, 0, 1) at (1.524, 0, 0)
component "Top" placed x (1, 0, 0) y (0, 1, 0) z (0, 0, 1) at (7.874, 0, 0)
component "middle ring" placed x (1, 0, 0) y (0, 1, 0) z (0, 0, 1) at (1.524, 0, 0)
component "Inner ring" placed x (1, 0, 0) y (0, 1, 0) z (0, 0, 1) at (1.524, 0, 0)
